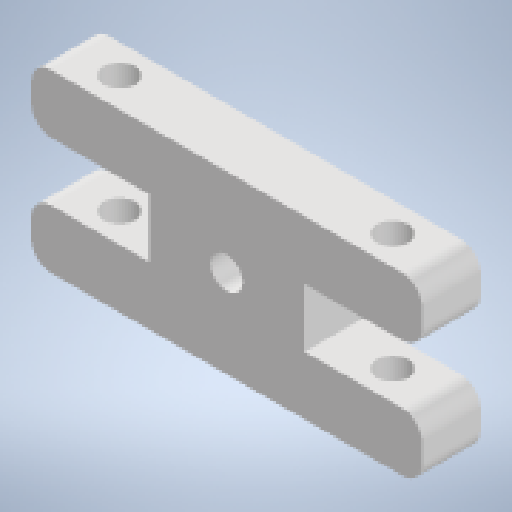
# Autodesk Inventor part: Connector
Saved by Autodesk Inventor 2023 (Build 270158000, 158)
## iProperties
Created: 2023-02-27
Part Number: Connector
Material: Generic
Document SubType Name: Modeling
Designer: Gabriel - T3 CAD
Density: 1 g/cm^3
Appearance: Default
Author: Gabriel - T3 CAD
Autodesk Inventor part; units mm, degrees
ref_plane "YZ Plane" through (0, 0, 0) normal (1, 0, 0) x (0, 1, 0)
ref_plane "XZ Plane" through (0, 0, 0) normal (0, 1, 0) x (-1, 0, 0)
ref_plane "XY Plane" through (0, 0, 0) normal (0, 0, 1) x (1, 0, 0)
sketch "Sketch1" plane through (0, 0, 0) normal (0, 0, 1) x (1, 0, 0)
  line L0 (0, 0) -> (-63.5, 0)
  line L1 (-63.5, 0) -> (-63.5, 28.575)
  line L2 (-63.5, 28.575) -> (0, 28.575)
  line L3 (0, 28.575) -> (0, 0)
  line L4 (0, 9.525) -> (-63.5, 9.525)
  line L5 (-63.5, 9.525) -> (-63.5, 19.05)
  line L6 (-63.5, 19.05) -> (0, 19.05)
  line L7 (0, 19.05) -> (0, 9.525)
  line L8 (-44.45, 28.575) -> (-19.05, 28.575)
  line L9 (-19.05, 28.575) -> (-19.05, 0)
  line L10 (-19.05, 0) -> (-44.45, 0)
  line L11 (-44.45, 0) -> (-44.45, 28.575)
  circle A0 centre (-31.75, 14.2875) radius 6.35
  circle A1 centre (-31.75, 14.2875) radius 2.5797
  point P0 (-19.05, 9.525)
  point P1 (-19.05, 19.05)
  point P2 (0, 19.05)
  point P3 (-44.45, 19.05)
  point P4 (-44.45, 9.525)
  dimension "d11" = 63.5
  dimension "d12" = 28.575
  dimension "d13" = 9.525
  dimension "d14" = 9.525
  dimension "d15" = 19.05
  dimension "d16" = 19.05
  dimension "d17" = 14.2875
  dimension "d18" = 31.75
  dimension "d19" = 12.7
  dimension "d20" = 5.1594
  constraints: 24 end point, 6 parallel, 4 point on line, 3 horizontal, 3 perpendicular, 2 centre point, 1 coincident
  measures "d11" distance of L0.start L0.end
  measures "d12" distance of L0.end L1.end
  measures "d13" distance between parallel lines of L0 L4
  measures "d14" distance between parallel lines of L6 L4
  measures "d15" distance between parallel lines of L1 L11
  measures "d16" distance between parallel lines of L3 L9
  measures "d17" distance from line of L10 A0.centre
  measures "d18" distance from line of L1 A0.centre
  measures "d19" diameter of A0
  measures "d20" diameter of A1
extrude "Extrusion1" add sketch "Sketch1" along normal blind 9.525 contours L0 L9 L4 L3 | L0 L11 L4 A0 L9 | L0 L1 L4 L11 | L4 A0 L6 L9 | L6 L9 L2 L3 | L11 L6 A0 L4 | A0 L4 | L4 A0 L6 | L6 A0 L11 L2 L9 | L6 L1 L2 L11 | L6 A0
extrude "Extrusion2" cut sketch "Sketch1" along normal blind 6.35 contours A0 L4 | L4 A0 L6 | L6 A0 | A1
sketch "Sketch2" plane through (-63.5, 28.575, 0) normal (0, 1, 0) x (1, 0, 0)
  circle A0 centre (53.975, -4.7625) radius 2.5797
  circle A1 centre (9.525, -4.7625) radius 2.5797
  line L0 (63.5, 0) -> (0, 0) projected
  line L1 (63.5, 0) -> (63.5, -9.525) projected
  line L2 (0, 0) -> (0, -9.525) projected
  dimension "d25" = 4.7625
  dimension "d26" = 4.7625
  dimension "d27" = 9.525
  dimension "d28" = 9.525
  dimension "d29" = 5.1594
  constraints: 2 centre point, 1 equal radius
  measures "d25" distance from line of L0 A0.centre
  measures "d26" distance from line of L0 A1.centre
  measures "d27" distance from line of L1 A0.centre
  measures "d28" distance from line of L2 A1.centre
  measures "d29" diameter of A0
extrude "Extrusion3" cut sketch "Sketch2" against normal through all
fillet "Fillet1" radius 3.175 8 edges at (0, 28.575, 4.7625) (0, 19.05, 4.7625) (0, 9.525, 4.7625) (0, 0, 4.7625) (-63.5, 28.575, 4.7625) (-63.5, 19.05, 4.7625) (-63.5, 9.525, 4.7625) (-63.5, 0, 4.7625)
equation "\"d13\" = 0.333333 * d12"
equation "\"d14\" = d13"
equation "\"d15\" = 2 * d13"
equation "\"d16\" = d15"
equation "\"d17\" = 0.5 * d12"
equation "\"d18\" = 0.5 * d11"
equation "\"d26\" = d25"
equation "\"d28\" = d27"
body "Solid1"
